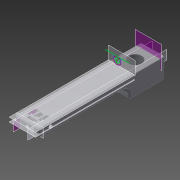
# Autodesk Inventor part: Link0
Saved by Autodesk Inventor 2015 (Build 190159000, 159)
## iProperties
Created: 2017-07-03
Part Number: Link0
Material: Generic
Document SubType Name: Modeling
Designer: Bruno
Density: 1 g/cm^3
Appearance: Default
Author: Bruno
Autodesk Inventor part; units mm, degrees
ref_plane "YZ Plane" through (0, 0, 0) normal (1, 0, 0) x (0, 1, 0)
ref_plane "XZ Plane" through (0, 0, 0) normal (0, 1, 0) x (-1, 0, 0)
ref_plane "XY Plane" through (0, 0, 0) normal (0, 0, 1) x (1, 0, 0)
sketch "Sketch1" plane through (0, 0, 0) normal (0, 0, 1) x (1, 0, 0)
  line L0 (0, 0) -> (0, 80)
  line L1 (0, 80) -> (0, 95)
  line L2 (0, 0) -> (0, -15)
  circle A0 centre (0, 80) radius 5.5
  line L3 (0, 80) -> (0, 72)
  line L4 (10, -10) -> (-10, -10)
  line L5 (10, 0) -> (10, -10)
  line L6 (-10, 0) -> (-10, -10)
  line L7 (-10.5, 80) -> (-5.5, 80)
  line L8 (10, 0) -> (10, 51.2877)
  line L9 (-10, 51.2877) -> (-10, 0)
  line L10 (-1.6, 2.1749) -> (-1.6, -2.1749)
  line L11 (1.6, -2.1749) -> (1.6, 2.1749)
  line L12 (1.6, 2.1749) -> (-1.6, -2.1749) construction
  line L13 (-1.6, 2.1749) -> (1.6, -2.1749) construction
  arc A1 (-1.6, -2.1749) -> (1.6, -2.1749) centre (0, 0) ccw
  arc A2 (1.6, 2.1749) -> (-1.6, 2.1749) centre (0, 0) ccw
  line L14 (10, 51.2877) -> (10, 95)
  line L15 (10, 95) -> (-10, 95)
  line L16 (-10, 95) -> (-10, 51.2877)
  point P0 (0, 40)
  dimension "d5" = 11
  dimension "d0" = 80
  dimension "d1" = 15
  dimension "d2" = 15
  dimension "d6" = 8
  dimension "d22" = 3.2
  constraints: 34 end point, 5 parallel, 4 point on circle, 4 vertical, 3 midpoint, 2 centre point, 2 coincident, 1 collinear, 1 horizontal alignment, 1 point on line, 2 other
  measures "d0" distance of L0.start L0.end
  measures "d1" distance of L0.end L1.end
  measures "d2" distance of L0.start L2.end
  measures "d6" distance of L3.start L3.end
  measures "d22" distance of L11.start L10.end
extrude "Extrusion1" add sketch "Sketch1" along normal blind 7 contours A2 L10 A1 L2 L4 L6 L9 L16 L7 A0 L0 | L0 A0 L1 L15 L14 L8 L5 L4 L2 A1 L11 A2 | L7 L16 L15 L1 A0
sketch "Sketch2" plane through (0, 0, 0) normal (0, 0, -1) x (-1, 0, 0)
  line L0 (1.6, 2.1749) -> (1.6, -2.1749) projected
  line L1 (-1.6, -2.6) -> (-1.6, 2.6) projected
  line L2 (-1.6, 2.6) -> (1.6, 2.6) projected
  line L3 (1.6, -2.6) -> (-1.6, -2.6) projected
  circle A0 centre (0, 0) radius 2.8
  dimension "d16" = 5.6
  constraints: 1 centre point, 1 coincident
  measures "d16" diameter of A0
extrude "Extrusion2" cut sketch "Sketch2" against normal blind 1 contours A0 L1 | L1 A0 L2 L3 | L3 A0 | A0 L2
ref_plane "Work Plane4" through (-6, -10, 0) normal (-1, 0, 0) x (0, 0, 1)
ref_plane "Work Plane5" through (6, -10, 0) normal (1, 0, 0) x (0, 0, -1)
sketch "Sketch15" plane through (-10, -10, 0) normal (-1, 0, 0) x (0, 0, 1)
  line L0 (1, 7.2) -> (1, 12.8) projected
  line L1 (1, 12.1749) -> (7, 12.1749) projected
  line L2 (1, 7.8251) -> (7, 7.8251) projected
  line L3 (1, 12.1749) -> (1, 7.8251) projected
  line L4 (1, 10) -> (4, 10)
  circle A0 centre (4, 10) radius 1.8
  point P0 (0, 10)
  dimension "d61" = 3
  dimension "d62" = 3.6
  constraints: 2 end point, 1 centre point, 1 coincident, 1 horizontal, 1 midpoint
  measures "d61" distance of L4.start L4.end
  measures "d62" diameter of A0
extrude "Extrusion13" cut sketch "Sketch15" against normal blind 8.5
sketch "Sketch18" plane through (10, -10, 0) normal (1, 0, 0) x (0, 0, -1)
  circle A0 centre (-4, 10) radius 1.8 projected
  point P0 (0, 10)
extrude "Extrusion14" cut sketch "Sketch18" against normal blind 8.5
sketch "Sketch19" plane through (-10, -10, 0) normal (0, -1, 0) x (1, 0, 0)
  line L0 (8.4, 1) -> (8.4, 7) projected
  line L1 (11.6, 1) -> (11.6, 7) projected
  line L2 (8.4, 1) -> (11.6, 1) projected
  line L3 (12.8, 1) -> (7.2, 1) projected
  line L4 (0, 7) -> (20, 7) projected
  line L5 (10, 7) -> (10, 4)
  line L6 (0, 0) -> (20, 0) projected
  circle A0 centre (10, 4) radius 1.8
  point P0 (10, 0)
  dimension "d67" = 3
  dimension "d68" = 3.6
  constraints: 2 end point, 1 centre point, 1 coincident, 1 midpoint, 1 perpendicular
  measures "d67" distance of L5.start L5.end
  measures "d68" diameter of A0
extrude "Extrusion15" cut sketch "Sketch19" against normal blind 8 contours A0 L0 | L0 A0 L1 | L1 A0
ref_plane "Work Plane6" through (-10, -7.4, 0) normal (0, -1, 0) x (1, 0, 0)
sketch "Sketch20" plane through (-6, -10, 0) normal (-1, 0, 0) x (0, 0, 1)
  circle A0 centre (4, 10) radius 1.8 projected
  circle A1 centre (4, 10) radius 3
  line L0 (7, 7.8251) -> (7, 12.1749) projected
  line L1 (7, 8.2679) -> (4, 6.5359)
  line L2 (4, 6.5359) -> (1, 8.2679)
  line L3 (1, 8.2679) -> (1, 11.7321)
  line L4 (1, 11.7321) -> (4, 13.4641)
  line L5 (4, 13.4641) -> (7, 11.7321)
  line L6 (7, 11.7321) -> (7, 8.2679)
  point P0 (0, 10)
  point P1 (7, 10)
  dimension "d72" = 6
  constraints: 12 end point, 2 coincident, 2 midpoint, 1 centre point, 13 other
  measures "d72" diameter of A1
extrude "Extrusion16" cut sketch "Sketch20" against normal blind 3
sketch "Sketch21" plane through (6, -10, 0) normal (1, 0, 0) x (0, 0, -1)
  circle A0 centre (-4, 10) radius 1.8 projected
  circle A1 centre (-4, 10) radius 3
  line L0 (-7, 0) -> (-7, 105) projected
  line L1 (-7, 11.7321) -> (-4, 13.4641)
  line L2 (-4, 13.4641) -> (-1, 11.7321)
  line L3 (-1, 11.7321) -> (-1, 8.2679)
  line L4 (-1, 8.2679) -> (-4, 6.5359)
  line L5 (-4, 6.5359) -> (-7, 8.2679)
  line L6 (-7, 8.2679) -> (-7, 11.7321)
  point P0 (0, 10)
  point P1 (-7, 10)
  constraints: 12 end point, 2 coincident, 1 horizontal alignment, 1 midpoint, 1 point on line, 1 vertical, 15 other
extrude "Extrusion17" cut sketch "Sketch21" against normal blind 3
sketch "Sketch22" plane through (-10, -7.4, 0) normal (0, -1, 0) x (1, 0, 0)
  circle A0 centre (10, 4) radius 1.8 projected
  circle A1 centre (10, 4) radius 3
  line L0 (20, 7) -> (0, 7) projected
  line L1 (11.7321, 7) -> (13.4641, 4)
  line L2 (13.4641, 4) -> (11.7321, 1)
  line L3 (11.7321, 1) -> (8.2679, 1)
  line L4 (8.2679, 1) -> (6.5359, 4)
  line L5 (6.5359, 4) -> (8.2679, 7)
  line L6 (8.2679, 7) -> (11.7321, 7)
  point P0 (10, 0)
  point P1 (10, 7)
  dimension "d77" = 6
  constraints: 12 end point, 2 coincident, 2 midpoint, 1 centre point, 13 other
  measures "d77" diameter of A1
extrude "Extrusion18" cut sketch "Sketch22" against normal blind 3
sketch "Sketch23" plane through (0, 0, 7) normal (0, 0, 1) x (1, 0, 0)
  line L0 (-6, 3.4641) -> (-3, 3.4641) projected
  line L1 (-6, 3.4641) -> (-6, 1.7321) projected
  line L2 (-6, -1.7321) -> (-6, 1.7321) projected
  line L3 (-6, -1.7321) -> (-6, -3.4641) projected
  line L4 (-6, -3.4641) -> (-3, -3.4641) projected
  line L5 (-3, -1.7321) -> (-3, -3.4641) projected
  line L6 (-3, 1.7321) -> (-3, -1.7321) projected
  line L7 (-3, 3.4641) -> (-3, 1.7321) projected
  line L8 (3, -1.7321) -> (3, 1.7321) projected
  line L9 (3, 1.7321) -> (3, 3.4641) projected
  line L10 (6, 3.4641) -> (3, 3.4641) projected
  line L11 (3, -3.4641) -> (3, -1.7321) projected
  line L12 (6, -3.4641) -> (3, -3.4641) projected
  line L13 (6, 1.7321) -> (6, 3.4641) projected
  line L14 (6, -3.4641) -> (6, -1.7321) projected
  line L15 (6, 1.7321) -> (6, -1.7321) projected
  line L16 (-1.7321, -4.4) -> (1.7321, -4.4) projected
  line L17 (-3.4641, -4.4) -> (-1.7321, -4.4) projected
  line L18 (-3.4641, -7.4) -> (-3.4641, -4.4) projected
  line L19 (-3.4641, -7.4) -> (-1.7321, -7.4) projected
  line L20 (1.7321, -7.4) -> (-1.7321, -7.4) projected
  line L21 (1.7321, -7.4) -> (3.4641, -7.4) projected
  line L22 (3.4641, -7.4) -> (3.4641, -4.4) projected
  line L23 (1.7321, -4.4) -> (3.4641, -4.4) projected
  point P0 (0, 0)
extrude "Extrusion19" cut sketch "Sketch23" against normal blind 3
sketch "Sketch24" plane through (0, 0, 7) normal (0, 0, 1) x (1, 0, 0)
  line L0 (-10, 95) -> (10, 95)
  line L1 (10, 95) -> (10, 65)
  line L2 (10, 65) -> (-10, 65)
  line L3 (-10, 65) -> (-10, 95)
  circle A0 centre (0, 80) radius 5.5 projected
  point P0 (0, 0)
  dimension "d82" = 20
  dimension "d83" = 30
  constraints: 8 end point, 2 parallel, 1 horizontal, 1 perpendicular
  measures "d82" distance of L1.end L2.end
  measures "d83" distance of L0.end L1.end
extrude "Extrusion20" add sketch "Sketch24" along normal blind 10
sketch "Sketch25" plane through (-10, 65, 7) normal (0, -1, 0) x (1, 0, 0)
  line L0 (20, 0) -> (0, 0) projected
  line L1 (20, 0) -> (20, 10) projected
  line L2 (0, 10) -> (20, 10) projected
  line L3 (0, 0) -> (0, 10) projected
  line L4 (10, 10) -> (10, 7)
  circle A0 centre (10, 7) radius 1.8
  point P0 (10, -7)
  dimension "d86" = 3
  dimension "d87" = 3.6
  constraints: 2 end point, 1 centre point, 1 coincident, 1 midpoint, 1 vertical
  measures "d86" distance of L4.start L4.end
  measures "d87" diameter of A0
extrude "Extrusion21" cut sketch "Sketch25" against normal blind 10 contours A0
sketch "Sketch26" plane through (-10, 95, 0) normal (0, 1, 0) x (1, 0, 0)
  spline S0 degree 2 poles (11.8, -14) (11.8, -17.1177) (9.1, -15.5588) (6.4, -14) (9.1, -12.4412) (11.8, -10.8823) (11.8, -14) knots 0 0 0 0.333333 0.333333 0.666667 0.666667 1 1 1 weights 1 0.5 1 0.5 1 0.5 1 projected
  point P0 (10, 0)
  constraints: 1 other
extrude "Extrusion22" cut sketch "Sketch26" against normal blind 10
ref_plane "Work Plane7" through (-10, 91, 0) normal (0, 1, 0) x (1, 0, 0)
sketch "Sketch27" plane through (-10, 91, 0) normal (0, 1, 0) x (1, 0, 0)
  spline S0 degree 8 poles (11.8, -14) (11.8, -13.7656) (11.7651, -13.5307) (11.6951, -13.3022) (11.5916, -13.086) (11.457, -12.8876) (11.2949, -12.712) (11.1096, -12.5635) (10.7033, -12.3263) (10.4811, -12.2377) (10.2466, -12.1831) (10.0058, -12.1641) (9.765, -12.1815) (9.5301, -12.2347) (9.3074, -12.3219) (8.8983, -12.5572) (8.711, -12.7056) (8.5471, -12.8816) (8.4109, -13.0807) (8.3062, -13.298) (8.2353, -13.5278) (8.2, -13.7642) (8.2, -14.2358) (8.2353, -14.4722) (8.3062, -14.702) (8.4109, -14.9193) (8.5471, -15.1184) (8.711, -15.2944) (8.8983, -15.4428) (9.306, -15.6773) (9.5272, -15.7642) (9.7603, -15.8174) (9.9995, -15.8354) (10.2386, -15.8175) (10.4718, -15.7645) (10.693, -15.6777) (11.101, -15.4434) (11.2885, -15.295) (11.4525, -15.119) (11.5888, -14.9198) (11.6937, -14.7024) (11.7646, -14.4724) (11.8, -14.236) (11.8, -14) knots 0 0 0 0 0 0 0 0 0 0.165934 0.165934 0.165934 0.165934 0.165934 0.165934 0.165934 0.333058 0.333058 0.333058 0.333058 0.333058 0.333058 0.333058 0.5 0.5 0.5 0.5 0.5 0.5 0.5 0.666942 0.666942 0.666942 0.666942 0.666942 0.666942 0.666942 0.832967 0.832967 0.832967 0.832967 0.832967 0.832967 0.832967 1 1 1 1 1 1 1 1 1 projected
  circle A0 centre (10, -14) radius 3
  line L0 (15.5, -17) -> (4.5, -17) projected
  line L1 (8.2679, -17) -> (6.5359, -14)
  line L2 (6.5359, -14) -> (8.2679, -11)
  line L3 (8.2679, -11) -> (11.7321, -11)
  line L4 (11.7321, -11) -> (13.4641, -14)
  line L5 (13.4641, -14) -> (11.7321, -17)
  line L6 (11.7321, -17) -> (8.2679, -17)
  point P0 (10, 0)
  point P1 (10, -17)
  constraints: 12 end point, 2 midpoint, 1 centre point, 1 coincident, 14 other
extrude "Extrusion23" cut sketch "Sketch27" against normal blind 3
ref_plane "Work Plane8" through (-10, 69, 7) normal (0, -1, 0) x (1, 0, 0)
sketch "Sketch28" plane through (-10, 69, 7) normal (0, -1, 0) x (1, 0, 0)
  circle A0 centre (10, 7) radius 1.8 projected
  line L0 (20, 0) -> (0, 0) projected
  line L1 (20, 0) -> (20, 10) projected
  line L2 (0, 10) -> (20, 10) projected
  line L3 (0, 0) -> (0, 10) projected
  line L4 (8.2679, 10) -> (6.5359, 7) projected
  line L5 (6.5359, 7) -> (8.2679, 4) projected
  line L6 (8.2679, 4) -> (11.7321, 4) projected
  line L7 (11.7321, 4) -> (13.4641, 7) projected
  line L8 (13.4641, 7) -> (11.7321, 10) projected
  line L9 (0, 10) -> (20, 10) projected
  line L10 (8.2679, 10) -> (11.7321, 10) projected
  point P0 (10, -7)
extrude "Extrusion24" cut sketch "Sketch28" against normal blind 3 contours L8 L7 L6 L5 L4 L2
sketch "Sketch29" plane through (0, 0, 17) normal (0, 0, 1) x (1, 0, 0)
  line L0 (-1.7321, 91) -> (-3.4641, 91) projected
  line L1 (-3.4641, 91) -> (-3.4641, 88) projected
  line L2 (-1.7321, 88) -> (-3.4641, 88) projected
  line L3 (1.7321, 88) -> (-1.7321, 88) projected
  line L4 (3.4641, 88) -> (1.7321, 88) projected
  line L5 (3.4641, 91) -> (3.4641, 88) projected
  line L6 (3.4641, 91) -> (1.7321, 91) projected
  line L7 (-1.7321, 91) -> (1.7321, 91) projected
  line L8 (-1.7321, 72) -> (1.7321, 72) projected
  line L9 (-3.4641, 72) -> (-1.7321, 72) projected
  line L10 (-3.4641, 69) -> (-3.4641, 72) projected
  line L11 (-1.7321, 69) -> (-3.4641, 69) projected
  line L12 (1.7321, 69) -> (-1.7321, 69) projected
  line L13 (3.4641, 69) -> (1.7321, 69) projected
  line L14 (3.4641, 69) -> (3.4641, 72) projected
  line L15 (1.7321, 72) -> (3.4641, 72) projected
  point P0 (0, 0)
extrude "Extrusion25" cut sketch "Sketch29" against normal blind 3
sketch "Sketch31" plane through (-10, 65, 7) normal (0, -1, 0) x (1, 0, 0)
  circle A0 centre (10, 7) radius 1.8 projected
  circle A1 centre (10, 7) radius 3
  line L0 (7, 7) -> (7, 10)
  line L1 (0, 10) -> (20, 10) projected
  line L2 (13, 10) -> (13, 7)
  point P0 (10, -7)
  dimension "d100" = 6
  constraints: 4 end point, 2 point on circle, 2 point on line, 1 centre point, 1 coincident, 1 tangent, 1 vertical
  measures "d100" diameter of A1
ref_plane "Work Plane9" through (0, 0, 3.5) normal (0, 0, 1) x (1, 0, 0)
mirror "Mirror1" about plane through (0, 0, 3.5) normal (0, 0, 1) of "Extrusion25", "Extrusion24", "Extrusion23", "Extrusion22", "Extrusion21", "Extrusion20"
ref_plane "Work Plane10" through (0, 0, 7) normal (0, 0, 1) x (1, 0, 0)
split "Split1" plane through (0, 0, 7) removes the side toward (0, 0, 1)
fillet "Fillet2" radius 0.6 6 edges at (10, 27.5, 7) (10, 80, 7) (0, 95, 7) (-10, 27.5, 7) (-10, 80, 7) (0, -10, 7)
fillet "Fillet3" radius 1.5 5 edges at (0, -10, 0) (0, 65, -10) (0, 95, -10) (10, 80, -10) (-10, 80, -10)
fillet "Fillet4" radius 5 1 edges at (0, 65, 0)
fillet "Fillet5" radius 1.5 20 edges at (10, 63.5355, -1.4645) (10, 65, -6.75) (9.5607, 65.4393, -9.5607) (10, -9.5607, 0.4393) (10, -10, 3.95) (9.8243, -9.8243, 6.8243) (10, 25.75, 0) (-10, -9.5607, 0.4393) (-10, -10, 3.95) (-9.8243, -9.8243, 6.8243) (-10, 63.5355, -1.4645) (-10, 65, -6.75) (-9.5607, 65.4393, -9.5607) (-10, 25.75, 0) (9.8243, 94.8243, 6.8243) (9.5607, 94.5607, -9.5607) (10, 95, -1.05) (-9.8243, 94.8243, 6.8243) (-9.5607, 94.5607, -9.5607) (-10, 95, -1.05)
body "Solid1"
